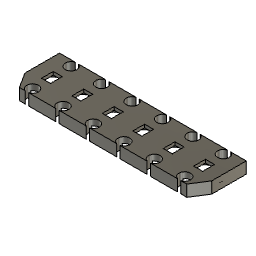
preset_block v6 (Autodesk Fusion 360 design; units mm, degrees)
Autodesk Fusion 360 part; units mm, degrees
sketch "Skizze1" plane through (0, 0, 0) normal (0, 0, 1) x (1, 0, 0)
  line L0 (67.5, -18) -> (-67.5, -18)
  line L1 (-67.5, -18) -> (-67.5, 18)
  line L2 (-67.5, 18) -> (67.5, 18)
  line L3 (67.5, 18) -> (67.5, -18)
  line L4 (67.5, -18) -> (-67.5, 18) construction
  line L5 (-67.5, -18) -> (67.5, 18) construction
  line L6 (-73.8697, 0) -> (79.3057, 0) construction
  line L7 (-75.373, 13.97) -> (76.9673, 13.97) construction
  line L8 (-75.54, -13.97) -> (74.2946, -13.97) construction
  line L9 (-11, 24.3178) -> (-11, -28.2997) construction
  line L10 (-33, 24.986) -> (-33, -31.4735) construction
  line L11 (-55, 24.4848) -> (-55, -28.1327) construction
  line L12 (11, 24.8189) -> (11, -31.4735) construction
  line L13 (33, 24.6519) -> (33, -30) construction
  line L14 (55, 24.8189) -> (55, -30) construction
  circle A0 centre (-55, 0) radius 12.2
  circle A1 centre (-33, 0) radius 12.2
  circle A2 centre (-11, 0) radius 12.2
  circle A3 centre (11, 0) radius 12.2
  circle A4 centre (33, 0) radius 12.2
  circle A5 centre (55, 0) radius 12.2
  circle A6 centre (-55, 13.97) radius 4.2
  circle A7 centre (-33, 13.97) radius 4.2
  circle A8 centre (-11, 13.97) radius 4.2
  circle A9 centre (11, 13.97) radius 4.2
  circle A10 centre (33, 13.97) radius 4.2
  circle A11 centre (55, 13.97) radius 4.2
  circle A12 centre (-55, -13.97) radius 4.2
  circle A13 centre (-33, -13.97) radius 4.2
  circle A14 centre (-11, -13.97) radius 4.2
  circle A15 centre (11, -13.97) radius 4.2
  circle A16 centre (33, -13.97) radius 4.2
  circle A17 centre (55, -13.97) radius 4.2
  circle A18 centre (-55, 0) radius 9.25
  circle A19 centre (-33, 0) radius 9.25
  circle A20 centre (-11, 0) radius 9.25
  circle A21 centre (11, 0) radius 9.25
  circle A22 centre (33, 0) radius 9.25
  circle A23 centre (55, 0) radius 9.25
  line L15 (-51.75, -4.25) -> (-58.25, -4.25)
  line L16 (-58.25, -4.25) -> (-58.25, 4.25)
  line L17 (-58.25, 4.25) -> (-51.75, 4.25)
  line L18 (-51.75, 4.25) -> (-51.75, -4.25)
  line L19 (-51.75, -4.25) -> (-58.25, 4.25) construction
  line L20 (-58.25, -4.25) -> (-51.75, 4.25) construction
  line L21 (-29.75, -4.25) -> (-36.25, -4.25)
  line L22 (-36.25, -4.25) -> (-36.25, 4.25)
  line L23 (-36.25, 4.25) -> (-29.75, 4.25)
  line L24 (-29.75, 4.25) -> (-29.75, -4.25)
  line L25 (-29.75, -4.25) -> (-36.25, 4.25) construction
  line L26 (-36.25, -4.25) -> (-29.75, 4.25) construction
  line L27 (-7.75, -4.25) -> (-14.25, -4.25)
  line L28 (-14.25, -4.25) -> (-14.25, 4.25)
  line L29 (-14.25, 4.25) -> (-7.75, 4.25)
  line L30 (-7.75, 4.25) -> (-7.75, -4.25)
  line L31 (-7.75, -4.25) -> (-14.25, 4.25) construction
  line L32 (-14.25, -4.25) -> (-7.75, 4.25) construction
  line L33 (14.25, -4.25) -> (7.75, -4.25)
  line L34 (7.75, -4.25) -> (7.75, 4.25)
  line L35 (7.75, 4.25) -> (14.25, 4.25)
  line L36 (14.25, 4.25) -> (14.25, -4.25)
  line L37 (14.25, -4.25) -> (7.75, 4.25) construction
  line L38 (7.75, -4.25) -> (14.25, 4.25) construction
  line L39 (36.25, -4.25) -> (29.75, -4.25)
  line L40 (29.75, -4.25) -> (29.75, 4.25)
  line L41 (29.75, 4.25) -> (36.25, 4.25)
  line L42 (36.25, 4.25) -> (36.25, -4.25)
  line L43 (36.25, -4.25) -> (29.75, 4.25) construction
  line L44 (29.75, -4.25) -> (36.25, 4.25) construction
  line L45 (58.25, -4.25) -> (51.75, -4.25)
  line L46 (51.75, -4.25) -> (51.75, 4.25)
  line L47 (51.75, 4.25) -> (58.25, 4.25)
  line L48 (58.25, 4.25) -> (58.25, -4.25)
  line L49 (58.25, -4.25) -> (51.75, 4.25) construction
  line L50 (51.75, -4.25) -> (58.25, 4.25) construction
  line L51 (-60.5, 33.1976) -> (-60.5, -30) construction
  line L52 (-89, -7) -> (78, -7) construction
  line L53 (-60.5, -18) -> (-67.5, -7)
  line L54 (60.5, 21.7982) -> (60.5, -34.2962) construction
  line L55 (60.5, -18) -> (67.5, -7)
  point P0 (-55, 0)
  point P1 (-33, 0)
  point P2 (-11, 0)
  point P3 (11, 0)
  point P4 (33, 0)
  point P5 (55, 0)
  dimension "d1" = 135
  dimension "d2" = 36
  dimension "d3" = 13.97
  dimension "d4" = 13.97
  dimension "d5" = 11
  dimension "d6" = 11
  dimension "d7" = 22
  dimension "d8" = 22
  dimension "d9" = 22
  dimension "d10" = 22
  dimension "d11" = 24.4
  dimension "d12" = 24.4
  dimension "d13" = 24.4
  dimension "d14" = 24.4
  dimension "d15" = 24.4
  dimension "d16" = 24.4
  dimension "d17" = 8.4
  dimension "d18" = 8.4
  dimension "d19" = 8.4
  dimension "d20" = 8.4
  dimension "d21" = 8.4
  dimension "d22" = 8.4
  dimension "d23" = 8.4
  dimension "d24" = 8.4
  dimension "d25" = 8.4
  dimension "d26" = 8.4
  dimension "d27" = 8.4
  dimension "d28" = 8.4
  dimension "d29" = 18.5
  dimension "d30" = 18.5
  dimension "d31" = 18.5
  dimension "d32" = 18.5
  dimension "d33" = 18.5
  dimension "d34" = 18.5
  dimension "d35" = 6.5
  dimension "d36" = 6.5
  dimension "d37" = 6.5
  dimension "d38" = 6.5
  dimension "d39" = 6.5
  dimension "d40" = 6.5
  dimension "d41" = 8.5
  dimension "d42" = 8.5
  dimension "d43" = 8.5
  dimension "d44" = 8.5
  dimension "d45" = 8.5
  dimension "d46" = 8.5
  dimension "d59" = 7
  dimension "d60" = 25
  dimension "d61" = 7
  dimension "d62" = 12.5
  dimension "d63" = 18
  constraint horizontal L0
  constraint perpendicular L0 L1
  constraint parallel L0 L2
  constraint parallel L1 L3
  constraint coincident L4 origin
  constraint coincident L5 origin
  constraint perpendicular L3 L6
  constraint perpendicular L1 L7
  constraint perpendicular L3 L8
  constraint perpendicular L0 L9
  constraint vertical L10
  constraint perpendicular L0 L11
  constraint perpendicular L2 L12
  constraint vertical L13
  constraint vertical L14
  constraint coincident L6 P0
  constraint coincident L11 P0
  constraint coincident L10 P1
  constraint coincident L6 P1
  constraint coincident L6 P2
  constraint coincident L9 P2
  constraint coincident L12 P3
  constraint coincident L6 P3
  constraint coincident L13 P4
  constraint coincident L6 P4
  constraint coincident L6 P5
  constraint coincident L14 P5
  constraint coincident L11 A6.centre
  constraint coincident L7 A6.centre
  constraint coincident L10 A7.centre
  constraint coincident L7 A7.centre
  constraint coincident L9 A8.centre
  constraint coincident L7 A8.centre
  constraint coincident L7 A9.centre
  constraint coincident L12 A9.centre
  constraint coincident L7 A10.centre
  constraint coincident L13 A10.centre
  constraint coincident L7 A11.centre
  constraint coincident L14 A11.centre
  constraint coincident L8 A12.centre
  constraint coincident L11 A12.centre
  constraint coincident L8 A13.centre
  constraint coincident L10 A13.centre
  constraint coincident L9 A14.centre
  constraint coincident L8 A14.centre
  constraint coincident L8 A15.centre
  constraint coincident L12 A15.centre
  constraint coincident L13 A16.centre
  constraint coincident L8 A16.centre
  constraint coincident L8 A17.centre
  constraint coincident L14 A17.centre
  constraint concentric A0 A18
  constraint concentric A1 A19
  constraint concentric A2 A20
  constraint concentric A3 A21
  constraint concentric A4 A22
  constraint concentric A5 A23
  constraint horizontal L15
  constraint perpendicular L15 L16
  constraint parallel L15 L17
  constraint parallel L16 L18
  constraint coincident L19 P0
  constraint coincident L20 P0
  constraint coincident P0 A0.centre
  constraint horizontal L21
  constraint perpendicular L21 L22
  constraint parallel L21 L23
  constraint parallel L22 L24
  constraint coincident L25 P1
  constraint coincident L26 P1
  constraint coincident P1 A1.centre
  constraint horizontal L27
  constraint perpendicular L27 L28
  constraint parallel L27 L29
  constraint parallel L28 L30
  constraint coincident L31 P2
  constraint coincident L32 P2
  constraint coincident P2 A2.centre
  constraint horizontal L33
  constraint perpendicular L33 L34
  constraint parallel L33 L35
  constraint parallel L34 L36
  constraint coincident L37 P3
  constraint coincident L38 P3
  constraint coincident P3 A3.centre
  constraint horizontal L39
  constraint perpendicular L39 L40
  constraint parallel L39 L41
  constraint parallel L40 L42
  constraint coincident L43 P4
  constraint coincident L44 P4
  constraint coincident P4 A4.centre
  constraint horizontal L45
  constraint perpendicular L45 L46
  constraint parallel L45 L47
  constraint parallel L46 L48
  constraint coincident L49 P5
  constraint coincident L50 P5
  constraint coincident P5 A5.centre
  constraint coincident origin L6
  constraint vertical L51
  constraint perpendicular L3 L52
  constraint coincident L51 L53.start
  constraint coincident L0 L53.start
  constraint coincident L1 L53.end
  constraint coincident L52 L53.end
  constraint perpendicular L7 L54
  constraint coincident L0 L55.start
  constraint coincident L54 L55.start
  constraint coincident L52 L55.end
  constraint coincident L3 L55.end
  measures "d1" distance of L1 L3
  measures "d2" distance of L0 L2
  measures "d3" distance of L6 L7
  measures "d4" distance of L6 L8
  measures "d5" distance of origin L12
  measures "d6" distance of origin L9
  measures "d7" distance of L12 L13
  measures "d8" distance of L13 L14
  measures "d9" distance of L9 L10
  measures "d10" distance of L10 L11
  measures "d11" diameter of A0
  measures "d12" diameter of A1
  measures "d13" diameter of A2
  measures "d14" diameter of A3
  measures "d15" diameter of A4
  measures "d16" diameter of A5
  measures "d17" diameter of A11
  measures "d18" diameter of A10
  measures "d19" diameter of A9
  measures "d20" diameter of A8
  measures "d21" diameter of A7
  measures "d22" diameter of A6
  measures "d23" diameter of A17
  measures "d24" diameter of A16
  measures "d25" diameter of A15
  measures "d26" diameter of A14
  measures "d27" diameter of A13
  measures "d28" diameter of A12
  measures "d29" diameter of A18
  measures "d30" diameter of A19
  measures "d31" diameter of A20
  measures "d32" diameter of A21
  measures "d33" diameter of A22
  measures "d34" diameter of A23
  measures "d35" distance of L16 L18
  measures "d36" distance of L22 L24
  measures "d37" distance of L28 L30
  measures "d38" distance of L34 L36
  measures "d39" distance of L40 L42
  measures "d40" distance of L46 L48
  measures "d41" distance of L45 L47
  measures "d42" distance of L39 L41
  measures "d43" distance of L33 L35
  measures "d44" distance of L27 L29
  measures "d45" distance of L21 L23
  measures "d46" distance of L15 L17
  measures "d59" distance of L1 L51
  measures "d60" distance of L2 L52
  measures "d61" distance of L3 L54
  measures "d62" distance of L1 A6.centre
  measures "d63" distance of L2 P0
extrude "Extrusion2" add sketch "Skizze1" along normal blind 8.3 contours L0 L2 L3 A5 A11 A17 L55 | L0 A5 A17 | L0 A4 A5 A16 A17 | L2 A5 A11 | L0 A4 A16 | A5 A17 | A4 A5 A11 A17 | L2 A4 A5 A10 A11 | L0 A3 A4 A15 A16 | A4 A5 | A3 A4 A5 A10 A16 | L2 A4 A10 | A5 A11 | L0 A3 A15 | A4 A16 | L2 A3 A4 A9 A10 | L0 A2 A3 A14 A15 | A3 A4 | A2 A3 A4 A9 A15 | A4 A10 | L2 A3 A9 | L0 A2 A14 | A3 A15 | L2 A2 A3 A8 A9 | L0 A1 A2 A13 A14 | A2 A3 | A1 A2 A3 A8 A14 | A3 A9 | L2 A2 A8 | L0 A1 A13 | A2 A14 | L2 A1 A2 A7 A8 | L0 A0 A1 A12 A13 | A1 A2 | A0 A1 A2 A7 A13 | A2 A8 | L2 A1 A7 | L0 A0 A12 | A1 A13 | L2 A0 A1 A6 A7 | L0 L1 L2 A0 A6 A12 L53 | A0 A1 | A0 A1 A6 A12 | A1 A7 | L2 A0 A6 | A0 A12 | A0 A6 | A18 | A19 | A20 | A21 | A22 | A23 | L15 L16 L17 L18 | L21 L22 L23 L24 | L27 L28 L29 L30 | L33 L34 L35 L36 | L39 L40 L41 L42 | L45 L46 L47 L48
extrude "Extrusion3" cut sketch "Skizze1" along normal blind 9 contours L0 A5 A17 | L2 A5 A11 | L0 A4 A16 | A5 A17 | L2 A4 A10 | A5 A11 | L0 A3 A15 | A4 A16 | A4 A10 | L2 A3 A9 | L0 A2 A14 | A3 A15 | A3 A9 | L2 A2 A8 | L0 A1 A13 | A2 A14 | A2 A8 | L2 A1 A7 | L0 A0 A12 | A1 A13 | A1 A7 | L2 A0 A6 | A0 A12 | A0 A6
extrude "Extrusion4" cut sketch "Skizze1" along normal blind 4 contours A4 A5 A11 A17 | A4 A5 | A3 A4 A5 A10 A16 | A3 A4 | A2 A3 A4 A9 A15 | A2 A3 | A1 A2 A3 A8 A14 | A1 A2 | A0 A1 A2 A7 A13 | A0 A1 | A0 A1 A6 A12
extrude "Extrusion5" cut sketch "Skizze1" along normal blind 6 contours A18 | A19 | A20 | A21 | A22 | A23
extrude "Extrusion6" cut sketch "Skizze1" along normal blind 9 contours L15 L16 L17 L18 | L21 L22 L23 L24 | L27 L28 L29 L30 | L33 L34 L35 L36 | L39 L40 L41 L42 | L45 L46 L47 L48
